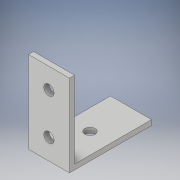
# Autodesk Inventor part: Bracket
Saved by Autodesk Inventor 2017 (Build 210142000, 142)
## iProperties
Created: 2018-07-12
Part Number: Bracket
Material: Generic
Document SubType Name: Modeling
Designer: sinner
Density: 1 g/cm^3
Appearance: Default
Author: sinner
Autodesk Inventor part; units mm, degrees
ref_plane "YZ Plane" through (0, 0, 0) normal (1, 0, 0) x (0, 1, 0)
ref_plane "XZ Plane" through (0, 0, 0) normal (0, 1, 0) x (-1, 0, 0)
ref_plane "XY Plane" through (0, 0, 0) normal (0, 0, 1) x (1, 0, 0)
sketch "Sketch1" plane through (0, 0, 0) normal (1, 0, 0) x (0, 1, 0)
  line L0 (0, 0) -> (50.8, 0)
  line L1 (50.8, 0) -> (50.8, -3.175)
  line L2 (3.175, -50.8) -> (0, -50.8)
  line L3 (0, -50.8) -> (0, 0)
  line L4 (3.175, -50.8) -> (3.175, -3.175)
  line L5 (3.175, -3.175) -> (50.8, -3.175)
  dimension "d0" = 3.175
  dimension "d1" = 50.8
  constraints: 12 end point, 4 perpendicular, 2 parallel, 1 horizontal, 1 vertical
  measures "d0" distance between parallel lines of L3 L4
  measures "d1" distance of L2.end L0.start
extrude "Extrusion1" add sketch "Sketch1" along normal blind 25.4
sketch "Sketch2" plane through (0, 3.175, -3.175) normal (0, 1, 0) x (1, 0, 0)
  line L0 (0, 47.625) -> (25.4, 47.625) projected
  line L1 (12.7, 47.625) -> (12.7, 13.7401) construction
  circle A0 centre (12.7, 22.225) radius 3.175
  line L2 (0, -3.175) -> (25.4, -3.175) projected
  dimension "d4" = 6.35
  dimension "d5" = 25.4
  constraints: 2 end point, 1 centre point, 1 midpoint, 1 point on line, 1 vertical
  measures "d4" diameter of A0
  measures "d5" distance from line of L2 A0.centre
extrude "Extrusion2" cut sketch "Sketch2" against normal blind 3.175
sketch "Sketch4" plane through (0, 3.175, -3.175) normal (0, 0, -1) x (-1, 0, 0)
  line L0 (0, 47.625) -> (-25.4, 47.625) projected
  line L1 (-12.7, 47.625) -> (-12.7, 26.8905) construction
  circle A0 centre (-12.7, 34.925) radius 3.175
  circle A1 centre (-12.7, 9.525) radius 3.175
  line L2 (0, -3.175) -> (-25.4, -3.175) projected
  dimension "d8" = 6.35
  dimension "d9" = 12.7
  dimension "d10" = 38.1
  constraints: 2 centre point, 2 end point, 2 point on line, 1 equal radius, 1 midpoint, 1 vertical
  measures "d8" diameter of A0
  measures "d9" distance from line of A1.centre L2
  measures "d10" distance from line of L2 A0.centre
extrude "Extrusion3" cut sketch "Sketch4" against normal blind 3.175
body "Solid1"
